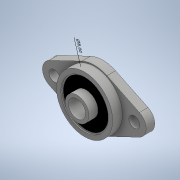
# Autodesk Inventor part: Kep Truc KLF-08
Saved by Autodesk Inventor 2021 (Build 250183000, 183)
## iProperties
Created: 2019-04-20
Part Number: Kep Truc KLF-08
Material: Generic
Document SubType Name: Modeling
Designer: Admin
Density: 1 g/cm^3
Appearance: Default(3)
Author: Admin
Autodesk Inventor part; units mm, degrees
ref_plane "YZ Plane" through (0, 0, 0) normal (1, 0, 0) x (0, 1, 0)
ref_plane "XZ Plane" through (0, 0, 0) normal (0, 1, 0) x (-1, 0, 0)
ref_plane "XY Plane" through (0, 0, 0) normal (0, 0, 1) x (1, 0, 0)
sketch "Sketch1" plane through (0, 0, 0) normal (0, 1, 0) x (-1, 0, 0)
  circle A0 centre (0, 0) radius 4
  arc A1 (-5.8378, -12.1725) -> (-5.8378, 12.1725) centre (0, 0) ccw
  circle A2 centre (18.5, 0) radius 2.5
  circle A3 centre (-18.5, 0) radius 2.5
  line L0 (0, -18.9) -> (0, 18.9) projected
  line L1 (20.8784, 4.9592) -> (5.8378, 12.1725)
  line L2 (33.6, 0) -> (-33.6, 0) projected
  line L3 (20.8784, -4.9592) -> (5.8378, -12.1725)
  line L4 (-20.8784, 4.9592) -> (-5.8378, 12.1725)
  line L5 (-20.8784, -4.9592) -> (-5.8378, -12.1725)
  arc A4 (-20.8784, 4.9592) -> (-20.8784, -4.9592) centre (-18.5, 0) ccw
  arc A5 (20.8784, -4.9592) -> (20.8784, 4.9592) centre (18.5, 0) ccw
  dimension "d0" = 8
  dimension "d1" = 27
  dimension "d2" = 5
  dimension "d3" = 5
  dimension "d4" = 37
  dimension "d5" = 18.5
  constraints: 8 end point, 8 point on circle, 6 centre point, 5 symmetric about line, 4 tangent, 3 coincident
  measures "d0" diameter of A0
  measures "d1" diameter of A1
  measures "d2" diameter of A2
  measures "d3" diameter of A3
  measures "d4" distance of A3.centre A2.centre
  measures "d5" distance of A2.centre point (0, 0)
extrude "Extrusion1" add sketch "Sketch1" along normal blind 4 contours L2 A1 L0 A0 | A0 L0 A1 L2 | A0 L2 A3 A4 L4 A1 L0 | L0 A1 L5 A4 L2 A3 A0 | L2 A2 A5 L3 A1 | A1 L1 A5 L2 A2
sketch "Sketch2" plane through (0, 0, 0) normal (0, -1, 0) x (1, 0, 0)
  circle A0 centre (0, 0) radius 4
  circle A1 centre (0, 0) radius 13
  dimension "d11" = 26
  constraints: 2 centre point, 2 coincident
  measures "d11" diameter of A1
extrude "Extrusion2" add sketch "Sketch2" along normal blind 4.5
sketch "Sketch3" plane through (0, -4.5, 0) normal (0, -1, 0) x (1, 0, 0)
  circle A0 centre (0, 0) radius 4
  circle A1 centre (0, 0) radius 4 projected
  circle A2 centre (0, 0) radius 5.5
  dimension "d14" = 11
  constraints: 2 centre point, 2 coincident
  measures "d14" diameter of A2
extrude "Extrusion3" add sketch "Sketch3" along normal blind 3.5
sketch "Sketch4" plane through (0, -4.5, 0) normal (0, -1, 0) x (1, 0, 0)
  circle A0 centre (0, 0) radius 5.5
  circle A1 centre (0, 0) radius 5.5 projected
  circle A2 centre (0, 0) radius 11
  dimension "d17" = 22
  constraints: 2 centre point, 2 coincident
  measures "d17" diameter of A2
extrude "Extrusion4" cut sketch "Sketch4" against normal blind 0.5
sketch "Sketch5" plane through (0, -4, 0) normal (0, -1, 0) x (1, 0, 0)
  circle A0 centre (0, 0) radius 5.5
  circle A1 centre (0, 0) radius 10.5
  dimension "d20" = 21
  constraints: 2 centre point, 2 coincident
  measures "d20" diameter of A1
extrude "Extrusion5" cut sketch "Sketch5" against normal blind 0.2
body "Solid1"
